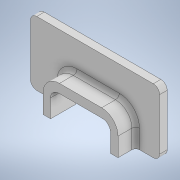
# Autodesk Inventor part: charge_support
Saved by Autodesk Inventor 2021 (Build 250183000, 183)
## iProperties
Created: 2024-06-07
Part Number: charge_support
Material: Generic
Document SubType Name: Modeling
Designer: Toby
Density: 1 g/cm^3
Appearance: Default
Author: Toby
Autodesk Inventor part; units mm, degrees
ref_plane "YZ Plane" through (0, 0, 0) normal (1, 0, 0) x (0, 1, 0)
ref_plane "XZ Plane" through (0, 0, 0) normal (0, 1, 0) x (-1, 0, 0)
ref_plane "XY Plane" through (0, 0, 0) normal (0, 0, 1) x (1, 0, 0)
sketch "Sketch1" plane through (0, 0, 0) normal (0, 0, 1) x (1, 0, 0)
  line L0 (-3.4123, 0.1305) -> (6.0877, 0.1305)
  line L1 (6.0877, 0.1305) -> (6.0877, -2.4395)
  line L2 (6.0877, -2.4395) -> (-3.4123, -2.4395)
  line L3 (-3.4123, -2.4395) -> (-3.4123, 0.1305)
  circle A0 centre (-2.1273, -1.1545) radius 1.285
  circle A1 centre (4.8027, -1.1545) radius 1.285
  line L4 (-4.6123, 1.5305) -> (7.2877, 1.5305)
  line L5 (7.2877, 1.5305) -> (7.2877, -2.4395)
  line L6 (7.2877, -2.4395) -> (-4.6123, -2.4395)
  line L7 (-4.6123, -2.4395) -> (-4.6123, 1.5305)
  point P0 (0, 0)
  point P1 (-3.4123, -2.4395)
  point P2 (-3.4123, -1.1545)
  point P3 (-2.1273, 0.1305)
  point P4 (4.8027, 0.1305)
  point P5 (6.0877, -1.1545)
  point P6 (6.0877, -2.4395)
  point P7 (4.8027, -2.4395)
  point P8 (-2.1273, -2.4395)
  dimension "d0" = 2.57
  dimension "d1" = 9.5
  dimension "d2" = 1.285
  dimension "d3" = 1.285
  dimension "d4" = 1.2
  dimension "d5" = 1.2
  dimension "d6" = 1.4
  constraints: 16 end point, 4 parallel, 2 centre point, 2 horizontal, 2 perpendicular, 2 tangent, 1 collinear
  measures "d0" distance between parallel lines of L2 L0
  measures "d1" distance of L0.start L0.end
  measures "d2" distance from line of L3 A0.centre
  measures "d3" distance from line of L1 A1.centre
  measures "d4" distance between parallel lines of L3 L7
  measures "d5" distance between parallel lines of L5 L1
  measures "d6" distance between parallel lines of L0 L4
extrude "Extrusion1" add sketch "Sketch1" along normal blind 4 contours L3 L6 L7 L4 L5 L1 L0 | L0 A0 L3 | L0 L1 A1
sketch "Sketch2" plane through (0, 0, 0) normal (0, 0, -1) x (-1, 0, 0)
  line L0 (-6.0877, -2.4395) -> (-7.2877, -2.4395) projected
  line L1 (-11.0877, 6.1305) -> (-6.6877, 6.1305)
  line L2 (-6.6877, 6.1305) -> (-6.6877, -2.4395)
  line L3 (-6.6877, -2.4395) -> (-11.0877, -2.4395)
  line L4 (-11.0877, -2.4395) -> (-11.0877, 6.1305)
  line L5 (4.6123, -2.4395) -> (3.4123, -2.4395) projected
  line L6 (4.0123, -2.4395) -> (9.4123, -2.4395)
  line L7 (9.4123, -2.4395) -> (9.4123, 6.1305)
  line L8 (9.4123, 6.1305) -> (4.0123, 6.1305)
  line L9 (4.0123, 6.1305) -> (4.0123, -2.4395)
  line L10 (-7.2877, 1.5305) -> (4.6123, 1.5305) projected
  line L11 (-6.6877, 6.1305) -> (4.0123, 6.1305)
  line L12 (4.0123, 6.1305) -> (4.0123, 1.5305)
  line L13 (4.0123, 1.5305) -> (-6.6877, 1.5305)
  line L14 (-6.6877, 1.5305) -> (-6.6877, 6.1305)
  line L15 (-6.0877, -1.1545) -> (-6.0877, -2.4395) projected
  line L16 (3.4123, -2.4395) -> (3.4123, -1.1545) projected
  line L17 (2.1273, 0.1305) -> (-4.8027, 0.1305) projected
  point P0 (0, 0)
  point P1 (-6.6877, 1.5305)
  point P2 (4.6123, -2.4395)
  dimension "d9" = 5
  dimension "d10" = 6
  dimension "d11" = 6
  constraints: 24 end point, 6 parallel, 3 horizontal, 3 perpendicular, 2 midpoint, 2 point on line, 1 collinear
  measures "d9" distance between parallel lines of L15 L4
  measures "d10" distance between parallel lines of L16 L7
  measures "d11" distance between parallel lines of L17 L11
extrude "Extrusion2" add sketch "Sketch2" against normal blind 1.2
fillet "Fillet1" radius 2.6 2 edges at (-4.6123, 1.5305, 2.6) (7.2877, 1.5305, 2.6)
sketch "Sketch3" plane through (-4.6123, -2.4395, 4) normal (0, -1, 0) x (1, 0, 0)
  line L0 (15.7, -2.8) -> (-4.8, -2.8) projected
  line L1 (1.2, -4) -> (1.2, 0) projected
  line L2 (-4.8, -2.8) -> (1.2, -2.8)
  line L3 (1.2, -2.8) -> (1.2, -4)
  line L4 (1.2, -4) -> (-4.8, -4)
  line L5 (-4.8, -4) -> (-4.8, -2.8)
  line L6 (0, -2.8) -> (0, 0) projected
  line L7 (0, 0) -> (1.2, 0)
  line L8 (1.2, 0) -> (1.2, -2.8)
  line L9 (1.2, -2.8) -> (0, -2.8)
  line L10 (0, -2.8) -> (0, 0)
  line L11 (11.9, -2.8) -> (11.9, 0) projected
  line L12 (10.7, -4) -> (10.7, 0) projected
  line L13 (11.9, 0) -> (10.7, 0)
  line L14 (10.7, 0) -> (10.7, -2.8)
  line L15 (10.7, -2.8) -> (11.9, -2.8)
  line L16 (11.9, -2.8) -> (11.9, 0)
  line L17 (15.7, -2.8) -> (10.7, -2.8)
  line L18 (10.7, -2.8) -> (10.7, -4)
  line L19 (10.7, -4) -> (15.7, -4)
  line L20 (15.7, -4) -> (15.7, -2.8)
  point P0 (4.6123, -4)
  point P1 (1.2, 0)
  constraints: 32 end point, 8 parallel, 4 horizontal, 4 perpendicular, 2 point on line
extrude "Extrusion3" add sketch "Sketch3" along normal blind 1.6
fillet "Fillet2" radius 0.6 5 edges at (6.5262, 0.769, 1.2) (1.3377, 1.5305, 1.2) (-3.8507, 0.769, 1.2) (-4.6123, -2.5545, 1.2) (7.2877, -2.5545, 1.2)
fillet "Fillet3" radius 1 4 edges at (-9.4123, -4.0395, 0.6) (-9.4123, 6.1305, 0.6) (11.0877, 6.1305, 0.6) (11.0877, -4.0395, 0.6)
body "Solid1"
